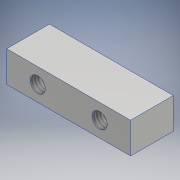
# Autodesk Inventor part: tap_straight_bottom
Saved by Autodesk Inventor 2018 (Build 220112000, 112)
## iProperties
Created: 2018-03-31
Part Number: tap_straight_bottom
Material: Aluminum 6061
Document SubType Name: Modeling
Designer: steve
Density: 2.7 g/cm^3
Appearance: Aluminum - Flat
Mass: 2.43182 g
Surface Area: 7.50285 cm^2
Volume: 0.900672 cm^3
Author: steve
Autodesk Inventor part; units mm, degrees
ref_plane "YZ Plane" through (0, 0, 0) normal (1, 0, 0) x (0, 1, 0)
ref_plane "XZ Plane" through (0, 0, 0) normal (0, 1, 0) x (-1, 0, 0)
ref_plane "XY Plane" through (0, 0, 0) normal (0, 0, 1) x (1, 0, 0)
sketch "Sketch1" plane through (0, 0, 0) normal (0, 0, 1) x (1, 0, 0)
  line L0 (-10, -3.45) -> (10, -3.45)
  line L1 (10, -3.45) -> (10, 3.45)
  line L2 (10, 3.45) -> (-10, 3.45)
  line L3 (-10, 3.45) -> (-10, -3.45)
  line L4 (-10, -3.45) -> (10, 3.45) construction
  line L5 (10, -3.45) -> (-10, 3.45) construction
  point P0 (0, 0)
  dimension "d0" = 20
  dimension "d1" = 6.9
  constraints: 12 end point, 2 midpoint, 2 parallel, 1 horizontal, 1 perpendicular
  measures "d0" distance between parallel lines of L1 L3
  measures "d1" distance of L0.end L1.end
extrude "Extrusion1" add sketch "Sketch1" along normal blind 5
sketch "Sketch2" plane through (-10, -3.45, 0) normal (0, -1, 0) x (1, 0, 0)
  line L0 (0, 0) -> (20, 0) construction
  line L1 (20, 0) -> (20, 5) construction
  line L2 (0, 5) -> (20, 5) construction
  line L3 (0, 0) -> (0, 5) construction
  line L4 (0, 2.5) -> (20, 2.5) construction
  line L5 (10, 0) -> (10, 9.5166) construction
  point P0 (5, 2.5)
  point P1 (15, 2.5)
  dimension "d4" = 5
  constraints: 4 end point, 2 midpoint, 1 point on line, 1 symmetric about line, 1 vertical
  measures "d4" distance from line of L5 point (5, 2.5)
hole "Hole1" at (-5, -3.45, 2.5) at (5, -3.45, 2.5) direction (0, 1, 0) diameter 2.459 depth 6 tip angle 118 thread size "M3x0.5" class "6H" standard "ISO Metric profile"
equation "\"d1\" = front_length"
equation "\"front_length\" = 6.9"
body "Solid1"
